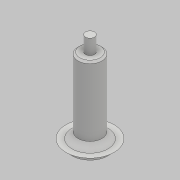
# Autodesk Inventor part: exercise2-2
Saved by Autodesk Inventor 2018 (Build 220112000, 112)
## iProperties
Created: 2020-09-19
Part Number: exercise2-2
Material: 一般
Document SubType Name: Modeling
Designer: 王鼎鈞
Density: 1 g/cm^3
Appearance: 預設
Author: 王鼎鈞
Autodesk Inventor part; units mm, degrees
ref_plane "YZ Plane" through (0, 0, 0) normal (1, 0, 0) x (0, 1, 0)
ref_plane "XZ Plane" through (0, 0, 0) normal (0, 1, 0) x (-1, 0, 0)
ref_plane "XY Plane" through (0, 0, 0) normal (0, 0, 1) x (1, 0, 0)
sketch "草圖1" plane through (0, 0, 0) normal (1, 0, 0) x (0, 1, 0)
  line L0 (-11.6463, 0) -> (69.8778, 0) projected
  line L1 (0, -192) -> (0, 32) projected
  line L2 (0, 0) -> (7.5, 0)
  line L3 (7.5, 0) -> (7.5, -25)
  line L4 (7.5, -25) -> (0, -25)
  line L5 (0, -25) -> (0, 0)
  line L6 (0, -25) -> (20, -25)
  line L7 (20, -25) -> (20, -140)
  line L8 (20, -140) -> (0, -140)
  line L9 (0, -140) -> (0, -25)
  line L10 (20, -140) -> (30, -150)
  line L11 (40, -150) -> (0, -150)
  line L12 (40, -150) -> (30, -160)
  line L13 (40, -150) -> (58.2315, -150) construction
  line L14 (0, -160) -> (30, -160)
  line L15 (0, -140) -> (0, -160)
  line L16 (30, -150) -> (20, -140)
  line L17 (30, -150) -> (0, -150)
  line L18 (20, -140) -> (0, -140)
  line L19 (0, -140) -> (0, -150)
  dimension "d0" = 7.5
  dimension "d1" = 25
  dimension "d2" = 20
  dimension "d4" = 140
  dimension "d5" = 135
  dimension "d6" = 10
  dimension "d7" = 40
  dimension "d8" = 0
  dimension "d9" = 135
  dimension "d11" = 160
  constraints: 36 end point, 4 horizontal, 4 parallel, 3 collinear, 3 perpendicular, 2 point on line
  measures "d0" distance of L3.end L4.end
  measures "d1" distance of L2.end L3.end
  measures "d2" distance of L7.end L8.end
  measures "d4" distance between parallel lines of L8 L0
  measures "d5" angle of L7 L10
  measures "d6" distance from line of L8 L10.end
  measures "d7" distance from line of L9 L11.start
  measures "d8" distance from line of L10.end L11
  measures "d9" angle of L12 L13
  measures "d11" distance between parallel lines of L2 L14
revolve "迴轉1" add sketch "草圖1" angle 360 about axis through (0, 0, -25) along (0, 0, 1)
chamfer "倒角1" distance 3 angle 45 1 edges at (0, -20, -25)
